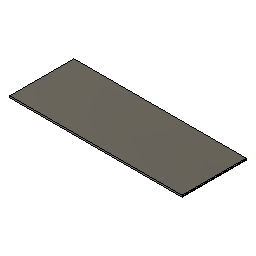
duct_panel (Autodesk Fusion 360 design; units mm, degrees)
part number: 2026-08-23-15-29-24-674
Autodesk Fusion 360 part; units mm, degrees
sketch "Panel outline" plane through (0, 0, 0) normal (0, 0, 1) x (1, 0, 0)
  line L0 (-97.22, 0) -> (97.22, 0)
  line L1 (97.22, 0) -> (97.22, 72)
  line L2 (97.22, 72) -> (-97.22, 72)
  line L3 (-97.22, 72) -> (-97.22, 0)
extrude "Panel" add sketch "Panel outline" along normal blind 2
chamfer "Groove lead-in" distance 0.6 angle 45 4 edges at (97.22, 36, 0) (97.22, 36, 2) (-97.22, 36, 0) (-97.22, 36, 2)
named bodies: "Duct Panel"
